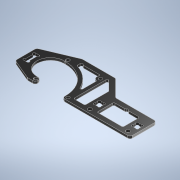
# Autodesk Inventor part: Ankle_side_frame
Saved by Autodesk Inventor 2022.3 (Build 263350000, 350)
## iProperties
Created: 2023-05-14
Part Number: Ankle_side_frame
Material: Generic
Document SubType Name: Modeling
Designer: Masato Kubotera
Density: 1 g/cm^3
Appearance: 光沢 - 黒
Description: A2017 T2
Mass: 2.45842 g
Surface Area: 37.8571 cm^2
Volume: 2.45842 cm^3
Author: Masato Kubotera
Revision Number: Rev.2 Specifications for RoboCup 2023: Changed shape of the actuator to make it easier to replace.
Autodesk Inventor part; units mm, degrees
ref_plane "YZ Plane" through (0, 0, 0) normal (1, 0, 0) x (0, 1, 0)
ref_plane "XZ Plane" through (0, 0, 0) normal (0, 1, 0) x (-1, 0, 0)
ref_plane "XY Plane" through (0, 0, 0) normal (0, 0, 1) x (1, 0, 0)
sketch "スケッチ1" plane through (0, 0, 0) normal (0, 1, 0) x (-1, 0, 0)
  line L0 (48, -16) -> (43, -16) construction
  line L1 (43, -16) -> (43, 6) construction
  line L2 (43, 6) -> (48, 6) construction
  line L3 (48, 6) -> (48, -16) construction
  line L4 (48, -16) -> (43, 6) construction
  line L5 (43, -16) -> (48, 6) construction
  line L6 (45.5, 6) -> (45.5, -16) construction
  line L7 (48, -7.5) -> (43, -7.5) construction
  line L8 (43, -7.5) -> (43, -2.5) construction
  line L9 (43, -2.5) -> (48, -2.5) construction
  line L10 (48, -2.5) -> (48, -7.5) construction
  line L11 (48, -7.5) -> (43, -2.5) construction
  line L12 (43, -7.5) -> (48, -2.5) construction
  line L13 (48.025, -7.525) -> (42.975, -7.525)
  line L14 (42.975, -7.525) -> (42.975, -2.475)
  line L15 (42.975, -2.475) -> (48.025, -2.475)
  line L16 (48.025, -2.475) -> (48.025, -7.525)
  line L17 (48.025, -7.525) -> (42.975, -2.475) construction
  line L18 (42.975, -7.525) -> (48.025, -2.475) construction
  line L19 (42.975, -5) -> (48.025, -5) construction
  arc A0 (44.4599, -2.475) -> (42.975, -3.9599) centre (43.7175, -3.2175) ccw
  arc A1 (48.025, -3.9599) -> (46.5401, -2.475) centre (47.2825, -3.2175) ccw
  arc A2 (42.975, -6.0401) -> (44.4599, -7.525) centre (43.7175, -6.7825) ccw
  arc A3 (46.5401, -7.525) -> (48.025, -6.0401) centre (47.2825, -6.7825) ccw
  circle A4 centre (0, 0) radius 10.5 construction
  line L20 (1, 13.5) -> (28, 13.5) construction
  line L21 (28, 13.5) -> (28, -13.5) construction
  line L22 (28, -13.5) -> (1, -13.5) construction
  line L23 (1, -13.5) -> (1, 13.5) construction
  line L24 (1, 13.5) -> (28, -13.5) construction
  line L25 (28, 13.5) -> (1, -13.5) construction
  circle A5 centre (28, 13.5) radius 1.35
  arc A6 (-0.35, 13) -> (2.35, 13) centre (1, 13) ccw
  line L26 (-0.35, 13) -> (-0.35, 13.5)
  line L27 (2.35, 13) -> (2.35, 13.5)
  arc A7 (2.35, 13.5) -> (-0.35, 13.5) centre (1, 13.5) ccw
  circle A8 centre (1, 13.5) radius 2.25 construction
  circle A9 centre (28, 13.5) radius 2.25 construction
  line L28 (1, 0) -> (28, 0) construction
  circle A10 centre (28, -13.5) radius 1.35
  arc A11 (2.35, -13) -> (-0.35, -13) centre (1, -13) ccw
  line L29 (-0.35, -13) -> (-0.35, -13.5)
  line L30 (2.35, -13) -> (2.35, -13.5)
  arc A12 (-0.35, -13.5) -> (2.35, -13.5) centre (1, -13.5) ccw
  circle A13 centre (1, -13.5) radius 2.25 construction
  circle A14 centre (28, -13.5) radius 2.25 construction
  line L31 (-17.5, -5) -> (-14.5, -5) construction
  line L32 (-14.5, -5) -> (-14.5, 5) construction
  line L33 (-14.5, 5) -> (-17.5, 5) construction
  line L34 (-17.5, 5) -> (-17.5, -5) construction
  line L35 (-17.5, -5) -> (-14.5, 5) construction
  line L36 (-14.5, -5) -> (-17.5, 5) construction
  line L37 (-14.475, -5.025) -> (-17.525, -5.025)
  line L38 (-17.525, -5.025) -> (-17.525, 5.025)
  line L39 (-17.525, 5.025) -> (-14.475, 5.025)
  line L40 (-14.475, 5.025) -> (-14.475, -5.025)
  line L41 (-14.475, -5.025) -> (-17.525, 5.025) construction
  line L42 (-17.525, -5.025) -> (-14.475, 5.025) construction
  arc A15 (-17.525, 5.025) -> (-17.525, 2.925) centre (-17.525, 3.975) ccw
  line L43 (-16, 5.025) -> (-16, -5.025) construction
  line L44 (-17.525, 0) -> (-14.475, 0) construction
  arc A16 (-14.475, 2.925) -> (-14.475, 5.025) centre (-14.475, 3.975) ccw
  arc A17 (-17.525, -2.925) -> (-17.525, -5.025) centre (-17.525, -3.975) ccw
  arc A18 (-14.475, -5.025) -> (-14.475, -2.925) centre (-14.475, -3.975) ccw
  arc A19 (0, 16) -> (-12, 10.583) centre (0, 0) ccw construction
  line L45 (-12, 10.583) -> (-12, -10.583) construction
  line L46 (0, 16) -> (31, 16) construction
  line L47 (31, 16) -> (31, -16) construction
  arc A20 (-12, -10.583) -> (0, -16) centre (0, 0) ccw construction
  line L48 (0, -16) -> (31, -16) construction
  circle A21 centre (45.5, -12.8) radius 1.6
  line L49 (82, -16) -> (82, 6)
  line L50 (82, 6) -> (48, 6)
  line L51 (48, 6) -> (34, 20)
  line L52 (34, 20) -> (6.2899, 20)
  line L53 (6.2899, 20) -> (-20.5, 8.739)
  line L54 (-20.5, 8.739) -> (-20.5, -8.739)
  line L55 (-20.5, -8.739) -> (-3.2261, -16)
  line L56 (-3.2261, -16) -> (3.25, -16)
  line L57 (3.25, -16) -> (3.25, -13.5)
  arc A22 (0, 11.25) -> (0, -11.25) centre (0, 0) ccw
  line L58 (0, 11.25) -> (1, 11.25)
  arc A23 (25.75, -13.5) -> (1, 11.25) centre (1, -13.5) ccw
  arc A24 (3.25, -13.5) -> (1, -11.25) centre (1, -13.5) ccw
  line L59 (1, -11.25) -> (0, -11.25)
  line L60 (25.75, -13.5) -> (25.75, -16)
  line L61 (25.75, -16) -> (82, -16)
  arc A25 (26.0957, -1.6564) -> (9.3752, 12.956) centre (1, -13.5) ccw
  line L62 (11.4091, 16) -> (24.2919, 16)
  line L63 (45, 6) -> (45, -16) construction
  line L64 (8.677, 13.9093) -> (8.677, 16)
  line L65 (9.677, 17) -> (9.677, 17)
  arc A26 (10.5431, 16.5) -> (11.4091, 16) centre (11.4091, 17) ccw
  arc A27 (10.5431, 16.5) -> (9.677, 17) centre (9.677, 16) ccw
  arc A28 (8.677, 13.9093) -> (9.3752, 12.956) centre (9.677, 13.9093) ccw
  arc A29 (9.677, 17) -> (8.677, 16) centre (9.677, 16) ccw
  arc A30 (26.0957, -1.6564) -> (28, -1.2296) centre (27, -1.2296) ccw
  arc A31 (25.2189, 14.625) -> (24.2919, 16) centre (24.2919, 15) ccw
  line L66 (32, 16) -> (31.9289, 16)
  line L67 (32.636, 15.7071) -> (40.2071, 8.136)
  line L68 (40.5, 7.4289) -> (40.5, -11)
  line L69 (39.5, -12) -> (32, -12)
  line L70 (77.5, 30) -> (45, 30) construction
  line L71 (45, 30) -> (45, -12) construction
  line L72 (45, -12) -> (77.5, -12) construction
  line L73 (77.5, -12) -> (77.5, 30) construction
  line L74 (77.5, 30) -> (45, -12) construction
  line L75 (45, 30) -> (77.5, -12) construction
  line L76 (61.25, 30) -> (61.25, -12) construction
  line L77 (74.475, -7.525) -> (79.525, -7.525)
  line L78 (79.525, -7.525) -> (79.525, -2.475)
  line L79 (79.525, -2.475) -> (74.475, -2.475)
  line L80 (74.475, -2.475) -> (74.475, -7.525)
  arc A32 (79.525, -3.9599) -> (78.0401, -2.475) centre (78.7825, -3.2175) ccw
  arc A33 (75.9599, -2.475) -> (74.475, -3.9599) centre (75.2175, -3.2175) ccw
  arc A34 (78.0401, -7.525) -> (79.525, -6.0401) centre (78.7825, -6.7825) ccw
  arc A35 (74.475, -6.0401) -> (75.9599, -7.525) centre (75.2175, -6.7825) ccw
  circle A36 centre (77, -12.8) radius 1.6
  line L81 (71, -12) -> (51.5, -12)
  line L82 (50.5, -11) -> (50.5, 1)
  line L83 (72, 1) -> (72, -11)
  line L84 (72, -12) -> (50.5, 2) construction
  line L85 (50.5, -12) -> (72, 2) construction
  line L86 (31, 15) -> (31, -11)
  arc A37 (32, 16) -> (31, 15) centre (32, 15) ccw
  arc A38 (31, 15) -> (31, 15) centre (32, 15) ccw
  arc A39 (31, -11) -> (32, -12) centre (32, -11) ccw
  arc A40 (39.5, -12) -> (40.5, -11) centre (39.5, -11) ccw
  arc A41 (40.5, 7.4289) -> (40.2071, 8.136) centre (39.5, 7.4289) ccw
  arc A42 (32.636, 15.7071) -> (31.9289, 16) centre (31.9289, 15) ccw
  arc A43 (51.5, 2) -> (50.5, 1) centre (51.5, 1) ccw
  arc A44 (50.5, -11) -> (51.5, -12) centre (51.5, -11) ccw
  arc A45 (71, -12) -> (72, -11) centre (71, -11) ccw
  arc A46 (72, 1) -> (71, 2) centre (71, 1) ccw
  line L87 (74.5, -16) -> (79.5, -16) construction
  line L88 (79.5, -16) -> (79.5, 6) construction
  line L89 (79.5, 6) -> (74.5, 6) construction
  line L90 (74.5, 6) -> (74.5, -16) construction
  line L91 (51.5, 2) -> (59.5179, 2)
  line L92 (62.9821, 2) -> (71, 2)
  arc A47 (61.25, 3) -> (60.384, 2.5) centre (61.25, 2) ccw
  arc A48 (62.116, 2.5) -> (61.25, 3) centre (61.25, 2) ccw
  arc A49 (59.5179, 2) -> (60.384, 2.5) centre (59.5179, 3) ccw
  arc A50 (62.116, 2.5) -> (62.9821, 2) centre (62.9821, 3) ccw
  line L93 (-14.5, -10) -> (-17.5, -10)
  line L94 (-17.5, -10) -> (-17.5, 10) construction
  line L95 (-17.5, 10) -> (-14.5, 10) construction
  line L96 (-14.5, 10) -> (-14.5, -10) construction
  line L97 (-14.5, -10) -> (-17.5, 10) construction
  line L98 (-17.5, -10) -> (-14.5, 10) construction
  line L99 (28, -1.2296) -> (28, 9.627)
  arc A51 (28, 9.627) -> (27.25, 10.5953) centre (27, 9.627) ccw
  arc A52 (25.2189, 14.625) -> (27.25, 10.5953) centre (28, 13.5) ccw
  point P0 (45.5, -5)
  point P1 (45.5, -5)
  point P2 (45.5, -5)
  point P3 (14.5, 0)
  point P4 (-16, 0)
  point P5 (48, -5)
  point P6 (-20.5, 0)
  point P7 (8.677, 17)
  point P8 (32.3431, 16)
  point P9 (40.5, 7.8431)
  point P10 (40.5, -12)
  point P11 (31, -12)
  point P12 (61.25, 9)
  point P13 (75.9599, -2.475)
  point P14 (78.0401, -7.525)
  point P15 (74.475, -6.0401)
  point P16 (74.475, -3.9599)
  point P17 (46.5401, -7.525)
  point P18 (44.4599, -7.525)
  point P19 (42.975, -6.0401)
  point P20 (46.5401, -2.475)
  point P21 (48.025, -3.9599)
  point P22 (48.025, -6.0401)
  point P23 (5.2762, 14.7617)
  point P24 (-14.475, -2.925)
  point P25 (61.25, -5)
  point P26 (60.25, 2)
  point P27 (62.25, 2)
  point P28 (45.5, -5)
  point P29 (45.5, -5)
  point P30 (31.9645, 15.9994)
  dimension "d0" = 5
  dimension "d1" = 22
  dimension "d2" = 5
  dimension "d3" = 1.05
  dimension "d5" = 0.025
  dimension "d6" = 0.025
  dimension "d14" = 21
  dimension "d15" = 27
  dimension "d16" = 27
  dimension "d17" = 2.7
  dimension "d19" = 0.5
  dimension "d21" = 4.5
  dimension "d22" = 1
  dimension "d23" = 3
  dimension "d24" = 10
  dimension "d25" = 1.05
  dimension "d26" = 0.025
  dimension "d27" = 0.025
  dimension "d28" = 16
  dimension "d29" = 12
  dimension "d30" = 2.5
  dimension "d31" = 5
  dimension "d32" = 3.2
  dimension "d34" = 3
  dimension "d35" = 45
  dimension "d36" = 3
  dimension "d37" = 3
  dimension "d40" = 1
  dimension "d42" = 32.5
  dimension "d43" = 42
  dimension "d47" = 4
  dimension "d48" = 2.5
  dimension "d49" = 2.5
  dimension "d51" = 1
  dimension "d53" = 4
  dimension "d54" = 1
  dimension "d55" = 4
  dimension "d57" = 2.5
  dimension "d59" = 22.799
  dimension "d60" = 4
  dimension "d61" = 1
  dimension "d62" = 1
  dimension "d64" = 45
  dimension "d65" = 4
  dimension "d66" = 1
  dimension "d67" = 20
  dimension "d68" = 7.8
  dimension "d69" = 31
  dimension "d70" = 3
  dimension "d71" = 4
  constraints: 201 end point, 93 point on circle, 52 centre point, 48 symmetric about line, 47 tangent, 40 point on line, 37 midpoint, 23 equal radius, 21 parallel, 16 perpendicular, 15 horizontal, 12 coincident, 10 collinear, 6 vertical, 2 concentric, 1 horizontal alignment, 20 other
  measures "d0" distance of L2.end L1.end
  measures "d1" distance of L0.end L1.end
  measures "d2" distance of L7.start L9.end
  measures "d3" radius of A0
  measures "d5" distance between parallel lines of L14 L8
  measures "d6" distance between parallel lines of L15 L9
  measures "d14" diameter of A4
  measures "d15" distance of L21.end L22.end
  measures "d16" distance of L20.end L21.end
  measures "d17" diameter of A5
  measures "d19" distance of A6.centre A7.centre
  measures "d21" diameter of A9
  measures "d22" distance of A4.centre L28.start
  measures "d23" distance of L33.end L32.end
  measures "d24" distance of L32.end L31.end
  measures "d25" radius of A15
  measures "d26" distance between parallel lines of L39 L33
  measures "d27" distance between parallel lines of L38 L34
  measures "d28" radius of A19
  measures "d29" distance from line of L45 A4.centre
  measures "d30" distance between parallel lines of L32 L45
  measures "d31" distance between parallel lines of L19 L28
  measures "d32" diameter of A21
  measures "d34" distance of L0.start L63.end
  measures "d35" distance from line of A4.centre L63
  measures "d36" radial gap between concentric circles of A23 A25
  measures "d37" distance between parallel lines of L54 L34
  measures "d40" radius of A26
  measures "d42" distance of L70.start L70.end
  measures "d43" distance of L72.end L70.start
  measures "d47" vertical distance of L60.end point (31, -12)
  measures "d48" distance between parallel lines of L68 L1
  measures "d49" distance between parallel lines of L82 L3
  measures "d51" radius of A37
  measures "d53" distance between parallel lines of L51 L67
  measures "d54" radius of A43
  measures "d55" distance between parallel lines of L0 L72
  measures "d57" distance between parallel lines of L49 L88
  measures "d59" angle of L52 L53
  measures "d60" distance between parallel lines of L91 L50
  measures "d61" radius of A49
  measures "d62" vertical distance of L91.end A47.start
  measures "d64" angle of L51 L2
  measures "d65" distance between parallel lines of L62 L52
  measures "d66" distance from line of L46 L65.start
  measures "d67" distance of L93.end L94.end
  measures "d68" distance of A21.centre point (45.5, -5)
  measures "d69" distance from line of point (0, 0) L47
  measures "d70" radius of A52
  measures "d71" distance edge to line of A29 L53
extrude "押し出し1" add sketch "スケッチ1" along normal blind 2 contours L61 L60 A23 L58 A22 L59 A24 L57 L56 L55 L54 L53 L52 L51 L50 L49 | A38 L67 A42
fillet "フィレット1" radius 2 10 edges at (20.5, 1, 8.739) (20.5, 1, -8.739) (-6.2899, 1, 20) (-34, 1, 20) (-3.25, 1, -16) (-25.75, 1, -16) (-48, 1, 6) (-82, 1, 6) (-82, 1, -16) (3.2261, 1, -16)
equation "\"d6\" = d5"
equation "\"d27\" = d26"
